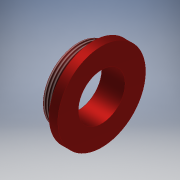
# Autodesk Inventor part: PayloadGermination_SyringeCap
Saved by Autodesk Inventor 2018 (Build 220112000, 112)
## iProperties
Created: 2018-07-29
Part Number: PayloadGermination_SyringeCap
Material: Aluminum 6061
Document SubType Name: Modeling
Designer: Bradley
Density: 2.7 g/cm^3
Appearance: Anodized - Red
Author: Bradley
Autodesk Inventor part; units mm, degrees
ref_plane "YZ Plane" through (0, 0, 0) normal (1, 0, 0) x (0, 1, 0)
ref_plane "XZ Plane" through (0, 0, 0) normal (0, 1, 0) x (-1, 0, 0)
ref_plane "XY Plane" through (0, 0, 0) normal (0, 0, 1) x (1, 0, 0)
sketch "Sketch1" plane through (0, 0, 0) normal (0, 1, 0) x (-1, 0, 0)
  line L0 (2, 4) -> (-2, 4)
  line L1 (-2, 4) -> (-2, 7.5)
  line L2 (-2, 7.5) -> (-0.5, 7.5)
  line L3 (-0.5, 7.5) -> (-0.5, 6)
  line L4 (-0.5, 6) -> (2, 6)
  line L5 (2, 6) -> (2, 4)
  line L6 (2, 0) -> (-2, 0)
  point P0 (0, 0)
  point P1 (0, 0)
  dimension "d0" = 15
  dimension "d1" = 1.5
  dimension "d2" = 12
  dimension "d3" = 2.5
  dimension "d4" = 8
  constraints: 14 end point, 5 perpendicular, 2 horizontal, 2 point on line, 1 coincident, 1 midpoint
  measures "d0" diameter of L2 L6
  measures "d1" distance of L1.end L2.end
  measures "d2" diameter of L4 L6
  measures "d3" distance of L3.end L4.end
  measures "d4" diameter of L0 L6
revolve "Revolution1" add sketch "Sketch1" angle 360 about axis through (-2, 0, 0) along (1, 0, 0)
thread "Thread1" size "M12x0.5" class "6g" standard "ANSI Metric M Profile" full length
body "Solid1"
